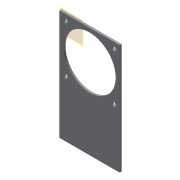
# Autodesk Inventor part: 200_Gearbox
Saved by Autodesk Inventor 2019 (Build 230136000, 136)
## iProperties
Created: 2019-07-08
Part Number: 200_Gearbox
Material: Generic
Document SubType Name: Modeling
Designer: diederichbenedict
Density: 1 g/cm^3
Appearance: Default
Author: diederichbenedict
Autodesk Inventor part; units mm, degrees
ref_plane "YZ Plane" through (0, 0, 0) normal (1, 0, 0) x (0, 1, 0)
ref_plane "XZ Plane" through (0, 0, 0) normal (0, 1, 0) x (-1, 0, 0)
ref_plane "XY Plane" through (0, 0, 0) normal (0, 0, 1) x (1, 0, 0)
ref_plane "Work Plane1" through (3.802, -31.8106, 0.3173) normal (0, 0, 1) x (1, 0.0036, 0)
sketch "Sketch4" plane through (3.802, -31.8106, 0.3173) normal (0, 0, 1) x (1, 0.0036, 0)
  circle A0 centre (23.8793, 0.0216) radius 1
  line L0 (26.85, -7.035) -> (26.8918, 3.0091)
  line L1 (26.8918, 3.0091) -> (16.8477, 3.0509)
  arc A1 (26.85, -7.035) -> (16.8477, 3.0509) centre (11.8295, -11.9283) ccw
  arc A2 (26.7284, -36.2501) -> (17.302, -26.7477) centre (11.8525, -41.5803) ccw
  circle A3 centre (23.7794, -23.9782) radius 1
  arc A4 (17.302, -26.7477) -> (26.8087, -16.9466) centre (11.8295, -11.9283) ccw
  arc A5 (26.7284, -36.2501) -> (17.302, -26.7477) centre (11.8525, -41.5803) ccw
  line L2 (26.7284, -36.2501) -> (26.8087, -16.9466)
  line L3 (23.1513, -51.9758) -> (26.3826, -51.9893)
  line L4 (26.3826, -51.9893) -> (26.4055, -46.4731)
  arc A6 (23.1513, -51.9758) -> (26.4055, -46.4731) centre (11.8525, -41.5803) ccw
  line L5 (-3.3369, -51.8656) -> (0.1141, -51.8799)
  arc A7 (-3.3097, -45.3197) -> (0.1141, -51.8799) centre (11.8525, -41.5803) ccw
  line L6 (-3.3097, -45.3197) -> (-3.3369, -51.8656)
  circle A8 centre (-0.2204, -23.8783) radius 1
  arc A9 (6.2945, -26.7245) -> (-3.2742, -36.8086) centre (11.8525, -41.5803) ccw
  arc A10 (-3.191, -16.8217) -> (6.2945, -26.7245) centre (11.8295, -11.9283) ccw
  line L7 (-3.191, -16.8217) -> (-3.2742, -36.8086)
  circle A11 centre (-0.1205, 0.1215) radius 1
  arc A12 (6.9361, 3.0922) -> (-3.1498, -6.9101) centre (11.8295, -11.9283) ccw
  line L8 (6.9361, 3.0922) -> (-3.108, 3.134)
  line L9 (-3.108, 3.134) -> (-3.1498, -6.9101)
  line L10 (26.85, -7.035) -> (26.8087, -16.9466)
  line L11 (-3.1498, -6.9101) -> (-3.191, -16.8217)
  line L12 (6.9361, 3.0922) -> (16.8477, 3.0509)
  line L13 (-3.2742, -36.8086) -> (-3.3097, -45.3197)
  line L14 (0.1141, -51.8799) -> (23.1513, -51.9758)
  line L15 (26.7284, -36.2501) -> (26.6628, -51.9904)
  line L16 (26.6628, -51.9904) -> (26.3826, -51.9893)
  circle A13 centre (11.8295, -11.9283) radius 13
  point P0 (-3.6879, 31.824)
extrude "Extrusion3" add sketch "Sketch4" along normal blind 1
body "Solid2"
